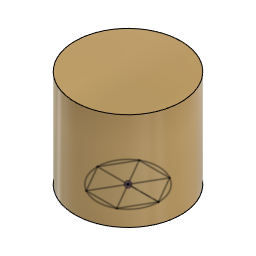
Stand Off Isolator (Printable) v5 (Autodesk Fusion 360 design; units mm, degrees)
Autodesk Fusion 360 part; units mm, degrees
sketch "post void" plane through (0, 0, 0) normal (0, 0, 1) x (1, 0, 0)
  circle A0 centre (0, 0) radius 3.75
  line L0 (0, 0) -> (1.875, 3.2476)
  line L1 (0, 0) -> (3.75, 0) construction
  line L2 (0, 0) -> (-1.875, 3.2476)
  line L3 (0, 0) -> (-3.75, 0)
  line L4 (0, 0) -> (-1.875, -3.2476)
  line L5 (0, 0) -> (1.875, -3.2476)
  line L6 (0, 0) -> (3.75, 0)
  line L7 (3.75, 0) -> (1.875, -3.2476)
  line L8 (1.875, -3.2476) -> (-1.875, -3.2476)
  line L9 (-1.875, -3.2476) -> (-3.75, 0)
  line L10 (-3.75, 0) -> (-1.875, 3.2476)
  line L11 (-1.875, 3.2476) -> (1.875, 3.2476)
  line L12 (1.875, 3.2476) -> (3.75, 0)
  dimension "d32" = 7.5
  dimension "d34" = 60
  dimension "d35" = 3.75
  dimension "d36" = 60
  dimension "d37" = 3.75
  dimension "d38" = 60
  dimension "d39" = 3.75
  dimension "d40" = 60
  dimension "d41" = 3.75
  dimension "d42" = 60
  dimension "d43" = 3.75
  dimension "d44" = 60
  dimension "d45" = 3.75
  constraint coincident A0.centre L0.start
  constraint horizontal L1
  constraint parallel L0 L7
  measures "d32" diameter of A0
  measures "d34" angle of L0 L1
  measures "d35" distance of A0.centre L0.end
  measures "d36" angle of L0 L2
  measures "d37" distance of A0.centre L2.end
  measures "d38" angle of L2 L3
  measures "d39" distance of A0.centre L3.end
  measures "d40" angle of L3 L4
  measures "d41" distance of A0.centre L4.end
  measures "d42" angle of L4 L5
  measures "d43" distance of A0.centre L5.end
  measures "d44" angle of L5 L6
  measures "d45" distance of A0.centre L1.end
sketch "Wall" plane through (0, 0, 0) normal (0, 0, 1) x (1, 0, 0)
  circle A0 centre (0, 0) radius 6.5
  dimension "d46" = 13
  constraint coincident A0.centre origin
  measures "d46" diameter of A0
extrude "Extrude1" add sketch "Wall" along normal blind 12
extrude "Extrude2" cut sketch "post void" along normal blind 8 contours L5 L6 L7 | L0 L6 L12 | L0 L2 L11 | L4 L5 L8 | L2 L3 L10 | L3 L4 L9
sketch "Sketch3" plane through (0, 0, 0) normal (0, 0, 1) x (1, 0, 0)
  circle A0 centre (0, 0) radius 1.9
  dimension "d51" = 3.8
  constraint coincident A0.centre origin
  measures "d51" diameter of A0
extrude "Extrude3" cut sketch "Sketch3" along normal blind 11
equation "d35 = ( 7.5 / 2 ) * 1 mm"
equation "d37 = ( 7.5 / 2 ) * 1 mm"
equation "d39 = ( 7.5 / 2 ) * 1 mm"
equation "d41 = ( 7.5 / 2 ) * 1 mm"
equation "d43 = ( 7.5 / 2 ) * 1 mm"
equation "d45 = ( 7.5 / 2 ) * 1 mm"
equation "d49 = 10.00 mm - 2 mm"
named bodies: "13mm"
